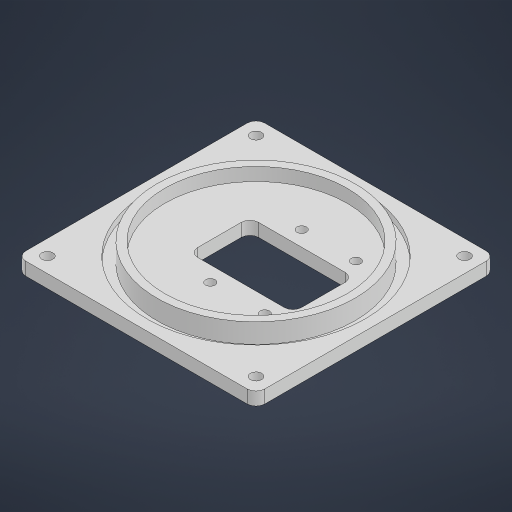
# Autodesk Inventor part: PiCameraMount
Saved by Autodesk Inventor 2024.2 (Build 282272000, 272)
## iProperties
Created: 2024-02-23
Part Number: PiCameraMount
Material: 一般
Document SubType Name: Modeling
Designer: Hanaoka
Density: 1 g/cm^3
Appearance: 既定
Author: Hanaoka
Autodesk Inventor part; units mm, degrees
ref_plane "YZ Plane" through (0, 0, 0) normal (1, 0, 0) x (0, 1, 0)
ref_plane "XZ Plane" through (0, 0, 0) normal (0, 1, 0) x (-1, 0, 0)
ref_plane "XY Plane" through (0, 0, 0) normal (0, 0, 1) x (1, 0, 0)
sketch "スケッチ1" plane through (0, 0, 0) normal (0, 1, 0) x (-1, 0, 0)
  line L0 (-25.5, 27.5) -> (25.5, 27.5)
  line L1 (27.5, 25.5) -> (27.5, -25.5)
  line L2 (25.5, -27.5) -> (-25.5, -27.5)
  line L3 (-27.5, -25.5) -> (-27.5, 25.5)
  line L4 (-27.5, 27.5) -> (27.5, -27.5) construction
  line L5 (27.5, 27.5) -> (-27.5, -27.5) construction
  arc A0 (27.5, 25.5) -> (25.5, 27.5) centre (25.5, 25.5) ccw
  arc A1 (-25.5, 27.5) -> (-27.5, 25.5) centre (-25.5, 25.5) ccw
  arc A2 (-27.5, -25.5) -> (-25.5, -27.5) centre (-25.5, -25.5) ccw
  arc A3 (25.5, -27.5) -> (27.5, -25.5) centre (25.5, -25.5) ccw
  line L6 (-24, -24) -> (24, -24) construction
  line L7 (24, -24) -> (24, 24) construction
  line L8 (24, 24) -> (-24, 24) construction
  line L9 (-24, 24) -> (-24, -24) construction
  line L10 (-24, -24) -> (24, 24) construction
  line L11 (24, -24) -> (-24, 24) construction
  circle A4 centre (24, 24) radius 1.3
  circle A5 centre (24, -24) radius 1.3
  circle A6 centre (-24, -24) radius 1.3
  circle A7 centre (-24, 24) radius 1.3
  point P0 (0, 0)
  dimension "d0" = 55
  dimension "d1" = 55
  dimension "d2" = 2
  dimension "d3" = 2.6
  dimension "d4" = 48
  constraints: 24 end point, 9 point on line, 8 centre point, 8 point on circle, 8 tangent, 6 equal radius, 4 coincident, 4 midpoint, 4 parallel, 2 horizontal, 2 perpendicular
  measures "d0" distance of L4.end L5.end
  measures "d1" distance of L5.end L4.start
  measures "d2" radius of A0
  measures "d3" diameter of A5
  measures "d4" distance of L8.end L6.start
extrude "押し出し1" add sketch "スケッチ1" along normal blind 3
sketch "スケッチ2" plane through (0, 3, 0) normal (0, 1, 0) x (1, 0, 0)
  line L0 (5.4, 5.4) -> (-5.4, 5.4)
  line L1 (-5.4, 5.4) -> (-5.4, -5.4) construction
  line L2 (-5.4, -5.4) -> (5.4, -5.4)
  line L3 (5.4, -5.4) -> (5.4, 5.4) construction
  line L4 (5.4, 5.4) -> (-5.4, -5.4) construction
  line L5 (-5.4, 5.4) -> (5.4, -5.4) construction
  circle A0 centre (0, 0) radius 2.875 construction
  line L6 (12.5, 10.5) -> (0, 10.5) construction
  line L7 (0, 10.5) -> (0, -10.5) construction
  line L8 (0, -10.5) -> (12.5, -10.5) construction
  line L9 (12.5, -10.5) -> (12.5, 10.5) construction
  line L10 (12.5, 10.5) -> (0, -10.5) construction
  line L11 (0, 10.5) -> (12.5, -10.5) construction
  circle A1 centre (0, -10.5) radius 1.1
  circle A2 centre (0, 10.5) radius 1.1
  circle A3 centre (12.5, 10.5) radius 1.1
  circle A4 centre (12.5, -10.5) radius 1.1
  line L12 (38.5, 0) -> (-38.5, 0) construction
  line L13 (-8.4, -7) -> (15.5, -7)
  line L14 (15.5, -7) -> (15.5, 7)
  line L15 (15.5, 7) -> (-8.4, 7)
  line L16 (-8.4, 7) -> (-8.4, -7)
  point P0 (6.25, 0)
  dimension "d8" = 10.8
  dimension "d9" = 10.8
  dimension "d10" = 5.75
  dimension "d11" = 2.2
  dimension "d12" = 21
  dimension "d13" = 12.5
  dimension "d14" = 14
  dimension "d15" = 3
  dimension "d16" = 3
  constraints: 32 end point, 6 parallel, 5 centre point, 5 midpoint, 4 coincident, 3 equal radius, 3 horizontal, 3 perpendicular, 1 point on line, 1 other
  measures "d8" distance of L2.end L0.start
  measures "d9" distance of L0.start L0.end
  measures "d10" diameter of A0
  measures "d11" diameter of A1
  measures "d12" distance of L6.end L7.end
  measures "d13" distance of L7.end L8.end
  measures "d14" distance of L15.end L13.start
  measures "d15" distance between parallel lines of L16 L1
  measures "d16" distance between parallel lines of L9 L14
extrude "押し出し2" cut sketch "スケッチ2" against normal up to surface (3 mm away)
fillet "フィレット1" radius 2 4 edges at (-8.4, 1.5, 7) (15.5, 1.5, 7) (15.5, 1.5, -7) (-8.4, 1.5, -7)
sketch "スケッチ3" plane through (0, 3, 0) normal (0, 1, 0) x (1, 0, 0)
  circle A0 centre (0, 0) radius 21
  circle A1 centre (0, 0) radius 22.8
  circle A2 centre (0, 0) radius 25.1
  dimension "d20" = 45.6
  dimension "d21" = 42
  dimension "d22" = 50.2
  constraints: 3 centre point, 3 coincident
  measures "d20" diameter of A1
  measures "d21" diameter of A0
  measures "d22" diameter of A2
extrude "押し出し3" add sketch "スケッチ3" along normal blind 3 contours A1
extrude "押し出し4" cut sketch "スケッチ3" against normal blind 1.5 contours A2
equation "\"d0\" = d1"
equation "\"d9\" = d8"
equation "\"d16\" = d15"
